Autodesk Inventor part; units mm, degrees
(part 2 of 2)
  spline S129 degree 2 poles (-17.2188, 91.866) (-17.0262, 92.076) (-16.5544, 92.5255) (-16.4136, 92.6564) knots 0 0 0 1 2 2 2
  line L146 (-16.4136, 92.6564) -> (-17.9104, 92.6564)
  line L147 (-17.9104, 92.6564) -> (-17.9104, 93.0096)
  spline S130 degree 2 poles (-20.1656, 92.0414) (-20.1656, 92.2612) (-20.0248, 92.6367) (-19.8963, 92.775) knots 0 0 0 1 2 2 2
  spline S131 degree 2 poles (-19.8963, 92.775) (-19.7679, 92.9133) (-19.385, 93.0738) (-19.1479, 93.0738) knots 0 0 0 1 2 2 2
  spline S132 degree 2 poles (-19.1479, 93.0738) (-18.9305, 93.0738) (-18.5057, 92.9775) (-18.3501, 92.9009) knots 0 0 0 1 2 2 2
  line L148 (-18.3501, 92.9009) -> (-18.3501, 92.4687)
  line L149 (-18.3501, 92.4687) -> (-18.3797, 92.4687)
  spline S133 degree 2 poles (-18.3797, 92.4687) (-18.4267, 92.5033) (-18.602, 92.5922) (-18.7082, 92.6317) knots 0 0 0 1 2 2 2
  spline S134 degree 2 poles (-18.7082, 92.6317) (-18.8293, 92.6737) (-19.0293, 92.7206) (-19.1553, 92.7206) knots 0 0 0 1 2 2 2
  spline S135 degree 2 poles (-19.1553, 92.7206) (-19.2788, 92.7206) (-19.511, 92.6317) (-19.595, 92.5354) knots 0 0 0 1 2 2 2
  spline S136 degree 2 poles (-19.595, 92.5354) (-19.6716, 92.444) (-19.7506, 92.2019) (-19.7506, 92.0389) knots 0 0 0 1 2 2 2
  spline S137 degree 2 poles (-19.7506, 92.0389) (-19.7506, 91.8759) (-19.6617, 91.6684) (-19.5777, 91.5992) knots 0 0 0 1 2 2 2
  spline S138 degree 2 poles (-19.5777, 91.5992) (-19.4912, 91.5227) (-19.2344, 91.4585) (-19.0787, 91.4585) knots 0 0 0 1 2 2 2
  spline S139 degree 2 poles (-19.0787, 91.4585) (-18.9108, 91.4585) (-18.5773, 91.5103) (-18.4761, 91.5326) knots 0 0 0 1 2 2 2
  line L150 (-18.4761, 91.5326) -> (-18.4761, 89.9616)
  line L151 (-18.4761, 89.9616) -> (-20.1483, 89.9616)
  line L152 (-20.1483, 89.9616) -> (-20.1483, 90.3198)
  line L153 (-20.1483, 90.3198) -> (-18.8688, 90.3198)
  line L154 (-18.8688, 90.3198) -> (-18.8688, 91.1324)
  spline S140 degree 2 poles (-18.8688, 91.1324) (-18.9429, 91.1225) (-19.0862, 91.1151) (-19.1454, 91.1151) knots 0 0 0 1 2 2 2
  spline S141 degree 2 poles (-19.1454, 91.1151) (-19.3801, 91.1151) (-19.7037, 91.1917) (-19.8519, 91.3053) knots 0 0 0 1 2 2 2
  spline S142 degree 2 poles (-19.8519, 91.3053) (-20.0025, 91.4189) (-20.1656, 91.7647) (-20.1656, 92.0414) knots 0 0 0 1 2 2 2
  point P0 (-47.5, 53.2457)
  constraints: 2 other
extrude "Extrusion47" cut sketch "Sketch58" against normal blind 1.5
sketch "Sketch59" plane through (69.5, 80.5, 0) normal (0, 0, -1) x (-1, 0, 0)
  line L0 (124.232, -148.2248) -> (124.232, -65.5994) projected
  line L1 (124.232, -131.7625) -> (22.225, -131.7625)
  line L2 (22.225, -144.4625) -> (124.232, -144.4625)
  line L3 (124.232, -144.4625) -> (124.232, -131.7625)
  line L4 (22.225, -144.4625) -> (19.05, -144.4625)
  line L5 (19.05, -144.4625) -> (19.05, -131.7625)
  line L6 (19.05, -131.7625) -> (22.225, -131.7625)
  point P0 (69.5, -80.5)
  point P1 (22.225, -131.7625)
  constraints: 12 end point, 2 horizontal, 2 parallel, 1 perpendicular, 1 point on line
extrude "Extrusion48" add sketch "Sketch59" against normal blind 1
sketch "Sketch61" plane through (-54.732, -66.7303, 5) normal (-1, 0, 0) x (0, 0, 1)
  point P0 (-5, 66.7303)
sketch "Sketch63" plane through (-54.732, -66.7303, 5) normal (-1, 0, 0) x (0, 0, 1)
  line L0 (0, 0) -> (32.8849, -46.9646) projected
  line L1 (32.8849, -46.9646) -> (72.2795, -19.3802)
  line L2 (72.2795, -19.3802) -> (86.4989, -39.6875)
  line L3 (86.4989, -39.6875) -> (32.8849, -46.9646)
  point P0 (-5, 66.7303)
  constraints: 6 end point, 2 perpendicular
extrude "Extrusion50" cut sketch "Sketch63" against normal blind 155.1
sketch "Sketch64" plane through (-54.732, -87.3593, 75.4961) normal (0, -0.819152, 0.5735764) x (1, 0, 0)
  line L0 (6, 0) -> (6, -45.9148) projected
  line L1 (0, -45.9148) -> (0, 21.0852) projected
  line L2 (0, 0) -> (0, -5)
  line L3 (0, -5) -> (3.5, -5)
  line L4 (3.5, -5) -> (0.6132, 0)
  line L5 (0, 0) -> (0, 0.5341)
  line L6 (0, 0.5341) -> (0.3049, 0.5341)
  line L7 (0.3049, 0.5341) -> (0.6312, -0.0311)
  line L8 (98.464, 0) -> (104.464, 0) projected
  line L9 (104.464, 0) -> (104.464, -5)
  line L10 (104.464, 21.0852) -> (104.464, -45.9148) projected
  line L11 (104.464, -5) -> (100.964, -5)
  line L12 (100.964, -5) -> (103.8508, 0)
  line L13 (103.8508, 0) -> (104.1591, 0.5341)
  line L14 (104.1591, 0.5341) -> (104.464, 0.5341)
  line L15 (104.464, 0.5341) -> (104.464, -0.2668)
  point P0 (0.6132, 0)
  dimension "d248" = 5
  dimension "d249" = 3.5
  dimension "d250" = 60
  dimension "d251" = 5
  dimension "d252" = 3.5
  dimension "d253" = 60
  constraints: 24 end point, 7 point on line, 2 horizontal, 2 perpendicular
  measures "d248" distance of L2.start L2.end
  measures "d249" distance of L2.end L3.end
  measures "d250" angle of L4 L3
  measures "d251" distance of L8.end L9.end
  measures "d252" distance of L9.end L11.end
  measures "d253" angle of L12 L11
extrude "Extrusion51" cut sketch "Sketch64" against normal blind 100.764
sketch "Sketch65" plane through (47.5, -63.2207, 2.5425) normal (0, -0.5735764, -0.819152) x (-1, 0, 0)
  circle A0 centre (74.6125, -57.15) radius 2 projected
  circle A1 centre (74.6125, -57.15) radius 5
  circle A2 centre (84.6125, -33.45) radius 2 projected
  circle A3 centre (84.6125, -33.45) radius 5
  circle A4 centre (64.6125, -33.45) radius 2 projected
  circle A5 centre (64.6125, -33.45) radius 5
  point P0 (47.5, 53.2457)
  dimension "d254" = 10
  dimension "d255" = 10
  dimension "d256" = 10
  constraints: 3 centre point, 3 coincident
  measures "d254" diameter of A1
  measures "d255" diameter of A3
  measures "d256" diameter of A5
extrude "Extrusion52" cut sketch "Sketch65" against normal blind 3 contours A1 | A2 | A3 | A4 | A5
sketch "Sketch66" plane through (-48.732, -55.8368, 7.1384) normal (0, 0.819152, -0.5735764) x (1, 0, 0)
  line L0 (42.232, 0) -> (42.232, -16) projected
  line L1 (0, 0) -> (42.232, 0) projected
  line L2 (0, -16) -> (0, 0)
  line L3 (0, 0) -> (42.232, 0)
  line L4 (42.232, 0) -> (42.232, -16)
  arc A0 (34.925, -16) -> (9.0575, -16) centre (21.9913, -30.5193) ccw projected
  arc A1 (34.925, -16) -> (9.0575, -16) centre (21.9913, -30.5193) ccw
  line L5 (42.232, -16) -> (34.925, -16)
  line L6 (9.0575, -16) -> (0, -16)
  point P0 (48.732, -26.1792)
  constraints: 10 end point, 4 point on circle, 3 parallel, 2 horizontal, 2 perpendicular, 1 centre point
extrude "Extrusion53" add sketch "Sketch66" along normal blind 2
sketch "Sketch67" plane through (47.5, -58.6321, 9.0958) normal (0, 0.5735764, 0.819152) x (1, 0, 0)
  line L0 (-96.232, 5.4125) -> (-96.232, 15.858) projected
  line L1 (-3.768, -61.6176) -> (-3.768, 39.1469) projected
  line L2 (-3.768, 5.4125) -> (-3.768, 15.875)
  line L3 (-3.768, 15.875) -> (-96.232, 15.875)
  line L4 (-96.232, 15.875) -> (-96.232, 5.4125)
  line L5 (-3.768, 10.6437) -> (-96.232, 10.6437)
  point P0 (-47.5, 53.2457)
  point P1 (-96.232, 15.858)
  point P2 (-3.768, 10.6437)
  constraints: 8 end point, 2 midpoint, 1 parallel, 1 point on line
extrude "Extrusion54" add sketch "Sketch67" along normal blind 50
sketch "Sketch70" plane through (-48.732, -45.6281, -0.0098) normal (0, 0.819152, -0.5735764) x (1, 0, 0)
  line L0 (92.464, -37.9148) -> (92.464, -50) projected
  line L1 (0, -0.0119) -> (0, -60) projected
  line L2 (92.464, -50) -> (0, -50)
  line L3 (0, -50) -> (0, -0.0119)
  line L4 (0, -0.0119) -> (92.464, -0.0119)
  line L5 (92.464, -0.0119) -> (92.464, -50)
  point P0 (48.732, -26.1792)
  point P1 (0, -50)
  constraints: 8 end point, 2 parallel, 1 horizontal, 1 perpendicular
extrude "Extrusion57" add sketch "Sketch70" along normal blind 10
sketch "Sketch72" plane through (47.5, -29.9533, 50.0534) normal (0, 0.5735764, 0.819152) x (1, 0, 0)
  line L0 (-96.232, 39.1469) -> (-96.232, -61.6176) projected
  line L1 (-3.768, 10.6437) -> (-3.768, 15.875) projected
  line L2 (-96.232, 25.875) -> (-3.768, 25.875)
  line L3 (-3.768, 25.875) -> (-3.768, 10.6437)
  line L4 (-3.768, 10.6437) -> (-96.232, 10.6438)
  line L5 (-96.232, 10.6438) -> (-96.232, 25.875)
  point P0 (-47.5, 53.2457)
  point P1 (-3.768, 25.875)
  point P2 (-3.768, 25.875)
  constraints: 8 end point, 2 parallel, 1 horizontal, 1 perpendicular
extrude "Extrusion59" add sketch "Sketch72" along normal blind 10
sketch "Sketch75" plane through (-48.732, -45.6212, 0) normal (-1, 0, 0) x (0, 0, 1)
  line L0 (0, 126.1212) -> (0, -24.1778) projected
  line L1 (0, 17.4625) -> (-11.1125, 17.4625)
  line L2 (-11.1125, 17.4625) -> (-11.1125, -14.2875)
  line L3 (-11.1125, -14.2875) -> (0, -14.2875)
  line L4 (0, -14.2875) -> (0, 17.4625)
  point P0 (0, 45.6212)
  point P1 (0, -14.2875)
  constraints: 8 end point, 2 parallel, 1 horizontal, 1 perpendicular, 1 point on line
extrude "Extrusion60" cut sketch "Sketch75" against normal through all
sketch "Sketch76" plane through (-48.732, -49.9133, 2.9908) normal (0, -0.819152, 0.5735764) x (1, 0, 0)
  circle A0 centre (71.464, 32) radius 18.5
  line L0 (92.464, 37.9148) -> (92.464, 0) projected
  line L1 (92.464, 0) -> (0, 0) projected
  point P0 (48.732, 26.1792)
  dimension "d279" = 37
  dimension "d280" = 21
  dimension "d281" = 32
  constraints: 1 centre point
  measures "d279" diameter of A0
  measures "d280" distance from line of L0 A0.centre
  measures "d281" distance from line of A0.centre L1
extrude "Extrusion61" cut sketch "Sketch76" against normal through all
sketch "Sketch77" plane through (-48.732, -37.4366, -5.7455) normal (0, 0.819152, -0.5735764) x (1, 0, 0)
  circle A0 centre (21.62, -30.5) radius 20
  line L0 (92.464, -7.014) -> (0, -7.014) projected
  line L1 (0, -60) -> (92.464, -60) projected
  line L2 (0, -7.014) -> (0, -60) projected
  point P0 (48.732, -26.1792)
  dimension "d284" = 40
  dimension "d287" = 29.5
  dimension "d288" = 21.62
  constraints: 1 centre point
  measures "d284" diameter of A0
  measures "d287" distance from line of L1 A0.centre
  measures "d288" distance from line of L2 A0.centre
extrude "Extrusion62" cut sketch "Sketch77" against normal blind 16
sketch "Sketch79" plane through (-6.5, -99.9044, 57.5273) normal (1, 0, 0) x (0, -0.5735764, -0.819152)
  line L0 (16, 67) -> (16, 0) projected
  line L1 (0, 67) -> (16, 67) projected
  line L2 (0, 67) -> (0, 0) projected
  line L3 (16, 0) -> (0, 0) projected
  point P0 (-10.1792, 114.8332)
extrude "Extrusion63" add sketch "Sketch79" along normal through all
sketch "Sketch80" plane through (-49.732, -111.9495, 40.3251) normal (0, -0.819152, 0.5735764) x (1, 0, 0)
  line L0 (93.464, 21) -> (93.464, -3) projected
  line L1 (1, 21) -> (93.464, 21) projected
  line L2 (1, -3) -> (1, 21) projected
  line L3 (1, -3) -> (20.3155, -3) projected
  line L4 (20.3155, -3) -> (20.3155, 0) projected
  line L5 (20.3155, 0) -> (24.9235, 0) projected
  line L6 (24.9235, 0) -> (24.9235, -3) projected
  line L7 (24.9235, -3) -> (93.464, -3) projected
  line L8 (20.3155, -3) -> (24.9235, -3)
  line L9 (97.232, -3.2766) -> (-2.768, -3.2766) projected
  point P0 (49.732, 31.1792)
  constraints: 2 end point, 1 parallel
extrude "Extrusion64" add sketch "Sketch80" along normal blind 5
sketch "Sketch81" plane through (47.5, -63.2207, 2.5425) normal (0, -0.5735764, -0.819152) x (-1, 0, 0)
  circle A0 centre (74.6125, -57.15) radius 2 projected
  circle A1 centre (74.6125, -57.15) radius 5.0201
  point P0 (47.5, 53.2457)
  constraints: 1 centre point, 1 coincident
extrude "Extrusion65" cut sketch "Sketch81" against normal blind 3
sketch "Sketch84" plane through (69.5, 80.5, 0) normal (0, 0, -1) x (-1, 0, 0)
  line L0 (25.768, -21.5352) -> (25.768, -113.9135) projected
  line L1 (118.232, -21.5352) -> (25.768, -21.5352) projected
  line L2 (118.232, -113.9135) -> (118.232, -21.5352) projected
  circle A0 centre (7, -127) radius 1.7294 projected
  circle A1 centre (7, -37) radius 1.7294 projected
  circle A2 centre (7, -82) radius 1.7294 projected
  circle A3 centre (92, -7) radius 1.7294 projected
  circle A4 centre (137, -127) radius 1.7294 projected
  circle A5 centre (137, -82) radius 1.7294 projected
  circle A6 centre (137, -37) radius 1.7294 projected
  circle A7 centre (52, -7) radius 1.7294 projected
  line L3 (0, -150.299) -> (0, 0) projected
  line L4 (0, -150.299) -> (144, -150.299) projected
  line L5 (144, 0) -> (144, -150.299) projected
  line L6 (0, 0) -> (144, 0) projected
  line L7 (25.768, -113.9135) -> (118.232, -113.9135) projected
  point P0 (69.5, -80.5)
extrude "Extrusion68" add sketch "Sketch84" along normal blind 5 contours L1 L2 L7 L0 | L3 L6 L5 L4
sketch "Sketch86" plane through (47.5, -63.2207, 2.5425) normal (0, -0.5735764, -0.819152) x (-1, 0, 0)
  line L0 (96.232, 2.6893) -> (3.768, 2.6893) projected
  line L1 (3.768, 2.6893) -> (3.768, 2.1006) projected
  line L2 (96.232, 2.1006) -> (3.768, 2.1006) projected
  line L3 (96.232, 2.1006) -> (96.232, 2.6893) projected
  point P0 (47.5, 53.2457)
extrude "Extrusion70" add sketch "Sketch86" along normal blind 0.5
sketch "Sketch88" plane through (-74.5, -69.799, 5) normal (0, -1, 0) x (1, 0, 0)
  line L0 (25.768, -10) -> (25.768, -4) projected
  line L1 (118.232, -10) -> (25.768, -10) projected
  line L2 (118.232, -4) -> (118.232, -10) projected
  line L3 (25.768, -4.75) -> (118.232, -4.75)
  point P0 (74.5, -5)
  point P1 (25.768, -5)
  point P2 (118.232, -5)
  dimension "d328" = 5.25
  constraints: 2 end point, 2 point on line, 1 perpendicular
  measures "d328" distance between parallel lines of L1 L3
extrude "Extrusion72" cut sketch "Sketch88" against normal blind 92.4694
sketch "Sketch89" plane through (-74.5, -69.799, 5) normal (0, -1, 0) x (1, 0, 0)
  line L0 (21.768, -4.75) -> (122.232, -4.75)
  line L1 (122.232, -4.75) -> (122.232, -9.25)
  line L2 (122.232, -9.25) -> (21.768, -9.25)
  line L3 (21.768, -9.25) -> (21.768, -4.75)
  line L4 (124.232, 0) -> (124.232, 32.8849) projected
  line L5 (19.768, 0) -> (19.768, 32.8849) projected
  line L6 (25.768, -4) -> (118.232, -4) projected
  point P0 (74.5, -5)
  point P1 (21.768, -7)
  dimension "d320" = 2
  dimension "d321" = 2
  dimension "d322" = 4.5
  dimension "d323" = 0.75
  constraints: 8 end point, 2 parallel, 1 horizontal, 1 midpoint, 1 perpendicular
  measures "d320" distance between parallel lines of L4 L1
  measures "d321" distance from line of point (21.768, -7) L5
  measures "d322" distance between parallel lines of L2 L0
  measures "d323" distance between parallel lines of L6 L0
extrude "Extrusion73" cut sketch "Sketch89" against normal blind 135
sketch "Sketch90" plane through (47.5, -49.4549, 22.2022) normal (0, 0.5735764, 0.819152) x (1, 0, 0)
  line L0 (-3.768, 5.4125) -> (-3.768, -61.6176) projected
  line L1 (-3.768, -61.6176) -> (-11.768, -61.6176)
  circle A0 centre (-11.768, -61.6176) radius 2
  circle A1 centre (-36.768, -61.6176) radius 2
  circle A2 centre (-11.768, -25.6176) radius 2
  circle A3 centre (-36.768, -25.6176) radius 2
  point P0 (-47.5, 53.2457)
  dimension "d331" = 8
  dimension "d332" = 4
  dimension "d333" = 4
  dimension "d334" = 25
  dimension "d335" = 4
  dimension "d336" = 36
  dimension "d337" = 4
  dimension "d338" = 25
  constraints: 4 centre point, 2 end point, 1 coincident, 1 horizontal
  measures "d331" distance of L0.end L1.end
  measures "d332" diameter of A0
  measures "d333" diameter of A1
  measures "d334" distance of A1.centre L1.end
  measures "d335" diameter of A2
  measures "d336" distance of A2.centre L1.end
  measures "d337" diameter of A3
  measures "d338" distance of A3.centre A2.centre
extrude "Extrusion74" cut sketch "Sketch90" against normal blind 92.4694
sketch "Sketch92" plane through (-48.732, -54.1985, 5.9913) normal (0, 0.819152, -0.5735764) x (1, 0, 0)
  circle A0 centre (71.4375, -29.5) radius 18
  line L0 (71.4375, -11.5) -> (81.7569, -11.5)
  line L1 (34.925, -16) -> (92.464, -16) projected
  point P0 (48.732, -26.1792)
  point P1 (82.464, -16)
  point P2 (59.5316, -16)
  point P3 (83.3434, -16)
  dimension "d341" = 36
  dimension "d342" = 4.5
  constraints: 2 end point, 1 horizontal, 3 other
  measures "d342" distance between parallel lines of L0 L1
extrude "Extrusion75" cut sketch "Sketch92" against normal blind 25
fillet "Fillet2" radius 2 4 edges at (34.6114, -55.2615, 26.268) (10.7996, -55.2615, 26.268) (-13.807, -53.4491, 24.999) (-39.6745, -53.4491, 24.999)
sketch "Sketch94" plane through (47.5, -63.2207, 2.5425) normal (0, -0.5735764, -0.819152) x (-1, 0, 0)
  circle A0 centre (36.768, -61.6176) radius 2 projected
  circle A1 centre (36.768, -61.6176) radius 3.5
  circle A2 centre (11.768, -61.6176) radius 2 projected
  circle A3 centre (11.768, -61.6176) radius 3.5
  circle A4 centre (36.768, -25.6176) radius 2 projected
  circle A5 centre (36.768, -25.6176) radius 3.5
  circle A6 centre (11.768, -25.6176) radius 2 projected
  circle A7 centre (11.768, -25.6176) radius 3.5
  point P0 (47.5, 53.2457)
  dimension "d347" = 7
  dimension "d348" = 7
  dimension "d349" = 7
  dimension "d351" = 7
  constraints: 4 centre point, 4 coincident
  measures "d347" diameter of A1
  measures "d348" diameter of A3
  measures "d349" diameter of A5
  measures "d351" diameter of A7
extrude "Extrusion76" cut sketch "Sketch94" against normal blind 3
sketch "Sketch95" plane through (43.732, -87.3593, 75.4961) normal (0, -0.819152, 0.5735764) x (1, 0, 0)
  line L0 (-97.8508, 0) -> (-94.964, -5) projected
  line L1 (-94.964, -5) -> (-98.464, -5) projected
  line L2 (-98.464, -45.9148) -> (-98.464, -5) projected
  line L3 (-98.464, -45.9148) -> (-92.464, -45.9148) projected
  line L4 (-92.464, -21.9148) -> (-92.464, -45.9148) projected
  line L5 (-92.464, 0) -> (-92.464, -21.9148) projected
  line L6 (-97.8508, 0) -> (-92.464, 0) projected
  line L7 (6, -5) -> (2.5, -5) projected
  line L8 (2.5, -5) -> (5.3868, 0) projected
  line L9 (0, 0) -> (5.3868, 0) projected
  line L10 (0, -21.9148) -> (0, 0) projected
  line L11 (0, -45.9148) -> (0, -21.9148) projected
  line L12 (0, -45.9148) -> (6, -45.9148) projected
  line L13 (6, -5) -> (6, -45.9148) projected
  point P0 (-43.732, -11.7356)
extrude "Extrusion77" add sketch "Sketch95" along normal blind 4.969
sketch "Sketch96" plane through (-54.732, -66.7303, 5) normal (-1, 0, 0) x (0, 0, 1)
  line L0 (8.6045, 59.0442) -> (69.2505, -27.5672) projected
  line L1 (73.054, -24.2935) -> (34.2888, -51.4372)
  line L2 (75.0678, -27.1695) -> (36.3025, -54.3132)
  line L3 (36.3025, -54.3132) -> (34.2888, -51.4372)
  line L4 (73.054, -24.2935) -> (73.4428, -24.0213)
  line L5 (73.4428, -24.0213) -> (75.1284, -26.4287)
  line L6 (75.1284, -26.4287) -> (75.0678, -27.1695)
  line L7 (69.2505, -27.5672) -> (35.7351, -51.0349) projected
  point P0 (-5, 66.7303)
  dimension "d356" = 0.5
  constraints: 12 end point, 3 perpendicular
  measures "d356" distance between parallel lines of L7 L1
extrude "Extrusion78" cut sketch "Sketch96" against normal through all
sketch "Sketch97" plane through (-52.732, 65.201, -4.25) normal (0, 0, 1) x (1, 0, 0)
  line L0 (96.464, -31.5144) -> (4, -31.5144) projected
  line L1 (4, -42.5306) -> (4, -135) projected
  line L2 (96.464, -31.5144) -> (4, -31.5144)
  line L3 (4, -31.5144) -> (4, -44.45)
  line L4 (4, -44.45) -> (96.464, -44.45)
  line L5 (96.464, -44.45) -> (96.464, -31.5144)
  point P0 (52.732, -65.201)
  constraints: 8 end point, 2 parallel, 1 horizontal, 1 perpendicular, 1 point on line
extrude "Extrusion79" cut sketch "Sketch97" against normal blind 10
sketch "Sketch98" plane through (69.5, 80.5, -5) normal (0, 0, -1) x (-1, 0, 0)
  line L0 (118.232, -21.8923) -> (25.768, -21.8923) projected
  line L1 (25.768, -46.8134) -> (25.768, -21.8923) projected
  line L2 (118.232, -113.7384) -> (118.232, -21.8923) projected
  line L3 (25.768, -46.8134) -> (118.232, -46.8134)
  line L4 (118.232, -46.8134) -> (118.232, -26.9875)
  line L5 (118.232, -26.9875) -> (25.768, -26.9875)
  line L6 (25.768, -26.9875) -> (25.768, -46.8134)
  point P0 (69.5, -80.5)
  point P1 (25.768, -26.9875)
  point P2 (118.232, -46.8134)
  constraints: 8 end point, 2 parallel, 1 horizontal, 1 perpendicular, 1 point on line
extrude "Extrusion80" cut sketch "Sketch98" against normal blind 10 contours L2 L3 L1 L5
sketch "Sketch99" plane through (-48.732, -4.8178, 17.7) normal (1, 0, 0) x (0, 0, -1)
  line L0 (12.7, 58.3303) -> (12.7, 56.6419) projected
  line L1 (13.8823, 58.3303) -> (12.7, 58.3303) projected
  line L2 (12.7, 56.6419) -> (13.8823, 58.3303)
  point P0 (17.7, 4.8178)
  constraints: 2 end point
extrude "Extrusion81" add sketch "Sketch99" along normal blind 92.464
chamfer "Chamfer3" distance 2 angle 45 2 edges at (-48.732, -9.2603, 47.7717) (43.732, -9.2603, 47.7717)
body "Solid1"
